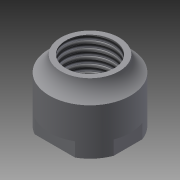
# Autodesk Inventor part: BallBearingCone
Saved by Autodesk Inventor 2015 (Build 190159000, 159)
## iProperties
Created: 2017-01-13
Part Number: BallBearingCone
Material: Generic
Document SubType Name: Modeling
Designer: 1esh9
Density: 1 g/cm^3
Appearance: Default
Author: 1esh9
Autodesk Inventor part; units mm, degrees
ref_plane "YZ Plane" through (0, 0, 0) normal (1, 0, 0) x (0, 1, 0)
ref_plane "XZ Plane" through (0, 0, 0) normal (0, 1, 0) x (-1, 0, 0)
ref_plane "XY Plane" through (0, 0, 0) normal (0, 0, 1) x (1, 0, 0)
sketch "Sketch1" plane through (0, 0, 0) normal (0, 0, 1) x (1, 0, 0)
  circle A0 centre (0, 0) radius 4.435
  circle A1 centre (0, 0) radius 7.46
  dimension "d0" = 8.87
  dimension "d1" = 14.92
  constraints: 2 centre point, 2 coincident
  measures "d0" diameter of A0
  measures "d1" diameter of A1
extrude "Extrusion1" add sketch "Sketch1" along normal blind 11.34
sketch "Sketch2" plane through (0, 0, 0) normal (0, 1, 0) x (-1, 0, 0)
  line L0 (7.46, 11.34) -> (-7.46, 11.34) projected
  line L1 (-7.46, 0) -> (7.46, 0) projected
  line L2 (7.46, 11.34) -> (-7.46, 11.34) projected
  line L3 (0, 11.34) -> (-5.375, 11.34) construction
  line L4 (-7.46, 0) -> (-7.46, 8.5) construction
  line L5 (-7.46, 0) -> (-7.46, 11.34) projected
  arc A0 (-7.46, 8.5) -> (-5.375, 11.34) centre (-9.3123, 12.0453) ccw
  line L6 (-5.375, 11.34) -> (-7.46, 11.34)
  line L7 (-7.46, 11.34) -> (-7.46, 8.5)
  line L8 (0, 11.34) -> (0, 0)
  dimension "d4" = 5.375
  dimension "d5" = 8.5
  dimension "d6" = 4
  constraints: 10 end point, 2 perpendicular, 2 point on circle, 2 point on line, 1 centre point, 1 collinear, 1 midpoint
  measures "d4" distance of L3.start L3.end
  measures "d5" distance of L1.start L4.end
  measures "d6" radius of A0
revolve "Revolution1" cut sketch "Sketch2" angle 360 about axis through (0, 0, 11.34) along (0, 0, -1) contours A0 L5 L0
thread "Thread1" size "M9x1.25" class "6H" standard "ANSI Metric M Profile" full length
sketch "Sketch3" plane through (0, 0, 0) normal (0, 0, -1) x (-1, 0, 0)
  circle A0 centre (0, 0) radius 4.435 projected
  circle A1 centre (0, 0) radius 7.46 projected
  line L0 (3.731, -6.46) -> (-3.731, -6.46)
  line L1 (3.731, 6.46) -> (-3.731, 6.46)
  line L2 (6.98, -2.6327) -> (6.98, 2.6327)
  line L3 (-6.98, -2.6327) -> (-6.98, 2.6327)
  dimension "d10" = 12.92
  dimension "d11" = 6.46
  dimension "d12" = 13.96
  dimension "d13" = 6.98
  constraints: 8 end point, 2 horizontal, 2 vertical, 9 other
  measures "d10" distance between parallel lines of L1 L0
  measures "d11" distance from line of point (0, 0) L1
  measures "d12" distance between parallel lines of L3 L2
  measures "d13" distance from line of point (0, 0) L2
extrude "Extrusion2" cut sketch "Sketch3" against normal blind 2.6 contours A1 L2 | L1 A1 | A1 L0 | L3 A1
equation "\"d11\" = 0.5 * d10"
equation "\"d13\" = 0.5 * d12"
body "Solid1"
